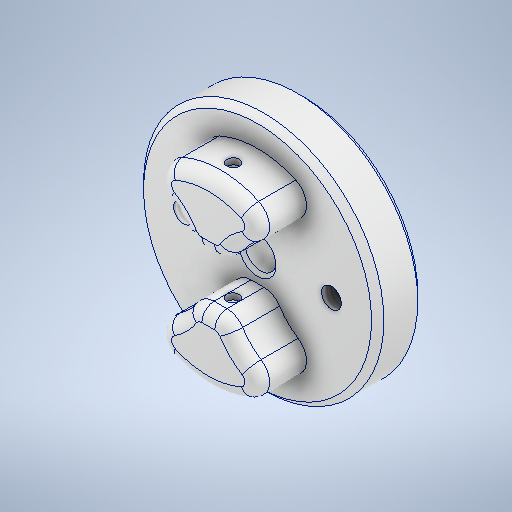
# Autodesk Inventor part: TorquimeterDisk
Saved by Autodesk Inventor 2025 (Build 290162000, 162)
## iProperties
Created: 2024-02-16
Part Number: TorquimeterDisk
Material: Aluminum 6061
Document SubType Name: Modeling
Designer: Vinicius
Density: 2.7 g/cm^3
Appearance: Aluminum - Flat
Mass: 20.646 g
Surface Area: 50.8443 cm^2
Volume: 7.64665 cm^3
Author: Vinicius
Autodesk Inventor part; units mm, degrees
ref_plane "YZ Plane" through (0, 0, 0) normal (1, 0, 0) x (0, 1, 0)
ref_plane "XZ Plane" through (0, 0, 0) normal (0, 1, 0) x (-1, 0, 0)
ref_plane "XY Plane" through (0, 0, 0) normal (0, 0, 1) x (1, 0, 0)
sketch "Sketch1" plane through (0, 0, 0) normal (0, 0, 1) x (1, 0, 0)
  circle A0 centre (0, 0) radius 19.5
  circle A1 centre (0, 0) radius 2.5
  dimension "d0" = 39
  dimension "d1" = 5
  constraints: 2 centre point, 2 coincident
  measures "d0" diameter of A0
  measures "d1" diameter of A1
extrude "Extrusion1" add sketch "Sketch1" along normal blind 7.5
sketch "Sketch2" plane through (0, 0, 7.5) normal (0, 0, 1) x (1, 0, 0)
  point P0 (0, 0)
  point P1 (12, 0)
  point P2 (-12, 0)
  dimension "d4" = 12
  dimension "d5" = 12
  constraints: 2 horizontal alignment
  measures "d4" distance of point (12, 0) point (0, 0)
  measures "d5" distance of point (-12, 0) point (0, 0)
hole "Hole1" at (12, 0, 7.5) at (-12, 0, 7.5) direction (0, 0, -1) diameter 3.242 end through all thread size "M4x0.7" class "6H" standard "ISO Metric profile"
chamfer "Chamfer1" distance 1 angle 45 1 edges at (-19.5, 0, 7.5)
sketch "Sketch5" plane through (0, 0, 7.5) normal (0, 0, 1) x (1, 0, 0)
  circle A0 centre (12, 0) radius 1.621 projected
  circle A1 centre (-12, 0) radius 1.621 projected
  circle A2 centre (12, 0) radius 10
  circle A3 centre (-12, 0) radius 10
  line L0 (2.8348, -4) -> (-2.8348, -4)
  line L1 (2.8348, 4) -> (-2.8348, 4)
  circle A4 centre (0, 0) radius 18.5 projected
  circle A5 centre (0, 0) radius 15
  arc A6 (6.1979, -13.6596) -> (6.5833, -8.4059) centre (4.9583, -10.9277) ccw
  arc A7 (-6.5833, -8.4059) -> (-6.1979, -13.6596) centre (-4.9583, -10.9277) ccw
  arc A8 (-1.0455, -4) -> (-3.5735, -5.3846) centre (-1.0455, -7) ccw
  arc A9 (3.5735, -5.3846) -> (1.0455, -4) centre (1.0455, -7) ccw
  point P0 (0, -4)
  point P1 (0, 4)
  dimension "d26" = 20
  dimension "d27" = 4
  dimension "d28" = 4
  dimension "d29" = 30
  dimension "d30" = 3
  dimension "d31" = 3
  constraints: 18 point on circle, 8 tangent, 7 centre point, 4 end point, 3 equal radius, 2 midpoint, 2 point on line, 1 coincident, 1 horizontal, 1 vertical alignment
  measures "d26" diameter of A3
  measures "d27" distance from line of L1 point (0, 0)
  measures "d28" distance of point (0, -4) point (0, 0)
  measures "d29" diameter of A5
  measures "d30" radius of A6
  measures "d31" radius of A9
extrude "Extrusion2" add sketch "Sketch5" along normal blind 8 contours A2 A6 A5 A7 A3 A8 L0 A9
pattern_circular "Circular Pattern1" count 2 over 360 about axis through (0, 0, 0) along (0, 0, 1) of "Extrusion2"
sketch "Sketch6" plane through (0, 0, 0) normal (0, 1, 0) x (-1, 0, 0)
  circle A0 centre (0, 11.5) radius 1
  line L0 (1.0455, 7.5) -> (1.0455, 15.5) projected
  point P0 (0, 0)
  point P1 (1.0455, 11.5)
  dimension "d37" = 2
  constraints: 1 centre point, 1 horizontal alignment, 1 midpoint, 1 vertical alignment
  measures "d37" diameter of A0
extrude "Extrusion3" cut sketch "Sketch6" along normal through all both and the other way through all
fillet "Fillet2" radius 2 16 edges at (-7.9503, 11.1472, 15.5) (-4.9155, 7.0576, 15.5) (-2.4867, 4.3688, 15.5) (0, 4, 15.5) (2.4867, 4.3688, 15.5) (4.9155, 7.0576, 15.5) (7.9503, 11.1472, 15.5) (0, 15, 15.5) (0, -4, 15.5) (-2.4867, -4.3688, 15.5) (-4.9155, -7.0576, 15.5) (-7.9503, -11.1472, 15.5) (0, -15, 15.5) (7.9503, -11.1472, 15.5) (4.9155, -7.0576, 15.5) (2.4867, -4.3688, 15.5)
sketch "Sketch7" plane through (0, 0, 0) normal (0, 0, -1) x (-1, 0, 0)
  arc A0 (1.0455, 4) -> (3.5735, 5.3846) centre (1.0455, 7) ccw projected
  arc A1 (6.5833, 8.4059) -> (3.5735, 5.3846) centre (12, 0) ccw projected
  arc A2 (6.5833, 8.4059) -> (6.1979, 13.6596) centre (4.9583, 10.9277) ccw projected
  arc A3 (6.1979, 13.6596) -> (-6.1979, 13.6596) centre (0, 0) ccw projected
  arc A4 (-6.1979, 13.6596) -> (-6.5833, 8.4059) centre (-4.9583, 10.9277) ccw projected
  arc A5 (-3.5735, 5.3846) -> (-6.5833, 8.4059) centre (-12, 0) ccw projected
  arc A6 (-3.5735, 5.3846) -> (-1.0455, 4) centre (-1.0455, 7) ccw projected
  line L0 (-1.0455, 4) -> (1.0455, 4) projected
  arc A7 (-1.0455, -4) -> (-3.5735, -5.3846) centre (-1.0455, -7) ccw projected
  arc A8 (-6.5833, -8.4059) -> (-3.5735, -5.3846) centre (-12, 0) ccw projected
  arc A9 (-6.5833, -8.4059) -> (-6.1979, -13.6596) centre (-4.9583, -10.9277) ccw projected
  arc A10 (-6.1979, -13.6596) -> (6.1979, -13.6596) centre (0, 0) ccw projected
  arc A11 (6.1979, -13.6596) -> (6.5833, -8.4059) centre (4.9583, -10.9277) ccw projected
  arc A12 (3.5735, -5.3846) -> (6.5833, -8.4059) centre (12, 0) ccw projected
  arc A13 (3.5735, -5.3846) -> (1.0455, -4) centre (1.0455, -7) ccw projected
  line L1 (1.0455, -4) -> (-1.0455, -4) projected
  circle A14 centre (0, 0) radius 2.5 projected
  circle A15 centre (12, 0) radius 1.621 projected
  circle A16 centre (-12, 0) radius 1.621 projected
  circle A17 centre (0, 0) radius 18.5 projected
  arc A18 (5.7847, 12.749) -> (-5.7847, 12.749) centre (0, 0) ccw
  arc A19 (6.0417, 9.2465) -> (5.7847, 12.749) centre (4.9583, 10.9277) ccw
  arc A20 (6.0417, 9.2465) -> (2.7308, 5.9231) centre (12, 0) ccw
  arc A21 (1.0455, 5) -> (2.7308, 5.9231) centre (1.0455, 7) ccw
  line L2 (1.0455, 5) -> (-1.0455, 5)
  arc A22 (-2.7308, 5.9231) -> (-1.0455, 5) centre (-1.0455, 7) ccw
  arc A23 (-2.7308, 5.9231) -> (-6.0417, 9.2465) centre (-12, 0) ccw
  arc A24 (-5.7847, 12.749) -> (-6.0417, 9.2465) centre (-4.9583, 10.9277) ccw
  arc A25 (-1.0455, -5) -> (-2.7308, -5.9231) centre (-1.0455, -7) ccw
  line L3 (-1.0455, -5) -> (1.0455, -5)
  arc A26 (2.7308, -5.9231) -> (1.0455, -5) centre (1.0455, -7) ccw
  arc A27 (2.7308, -5.9231) -> (6.0417, -9.2465) centre (12, 0) ccw
  arc A28 (5.7847, -12.749) -> (6.0417, -9.2465) centre (4.9583, -10.9277) ccw
  arc A29 (-5.7847, -12.749) -> (5.7847, -12.749) centre (0, 0) ccw
  arc A30 (-6.0417, -9.2465) -> (-5.7847, -12.749) centre (-4.9583, -10.9277) ccw
  arc A31 (-6.0417, -9.2465) -> (-2.7308, -5.9231) centre (-12, 0) ccw
  line L4 (-4.207, 7.7633) -> (4.207, 7.7633)
  line L5 (-4.207, -7.7633) -> (4.207, -7.7633)
  line L6 (-1.0455, 4) -> (-1.0455, 6) projected
  dimension "d41" = 1
  dimension "d42" = 1
  constraints: 32 point on circle, 14 centre point, 8 end point, 1 perpendicular, 14 other
  measures "d41" radial gap between concentric circles of A3 A18
  measures "d42" radial gap between concentric circles of A7 A25
extrude "Extrusion4" cut sketch "Sketch7" against normal blind 14 contours A22 A23 L4 A20 A21 L2 | A23 A24 A18 A19 A20 L4 | L3 A26 A27 L5 A31 A25 | L5 A27 A28 A29 A30 A31
sketch "Sketch8" plane through (0, 0, 0) normal (0, 0, -1) x (-1, 0, 0)
  arc A0 (2.7308, -5.9231) -> (6.0417, -9.2465) centre (12, 0) ccw projected
  arc A1 (5.7847, -12.749) -> (6.0417, -9.2465) centre (4.9583, -10.9277) ccw projected
  arc A2 (-5.7847, -12.749) -> (5.7847, -12.749) centre (0, 0) ccw projected
  arc A3 (-6.0417, -9.2465) -> (-5.7847, -12.749) centre (-4.9583, -10.9277) ccw projected
  arc A4 (-6.0417, -9.2465) -> (-2.7308, -5.9231) centre (-12, 0) ccw projected
  arc A5 (-2.7308, 5.9231) -> (-6.0417, 9.2465) centre (-12, 0) ccw projected
  arc A6 (-5.7847, 12.749) -> (-6.0417, 9.2465) centre (-4.9583, 10.9277) ccw projected
  arc A7 (5.7847, 12.749) -> (-5.7847, 12.749) centre (0, 0) ccw projected
  arc A8 (6.0417, 9.2465) -> (5.7847, 12.749) centre (4.9583, 10.9277) ccw projected
  arc A9 (6.0417, 9.2465) -> (2.7308, 5.9231) centre (12, 0) ccw projected
  circle A10 centre (-12, 0) radius 1.621 projected
  circle A11 centre (12, 0) radius 1.621 projected
  circle A12 centre (0, 0) radius 19.5 projected
  circle A13 centre (0, 0) radius 2.5 projected
  circle A14 centre (0, 0) radius 5
  circle A15 centre (0, 0) radius 8.83
  arc A16 (-4.207, 7.7633) -> (-6.0417, 9.2465) centre (-12, 0) ccw projected
  arc A17 (-5.8433, 6.62) -> (-6.0417, 9.2465) centre (-6.9363, 7.8582) ccw
  arc A18 (6.0417, 9.2465) -> (4.207, 7.7633) centre (12, 0) ccw projected
  arc A19 (6.0417, 9.2465) -> (5.8433, 6.62) centre (6.9363, 7.8582) ccw
  arc A20 (-6.0417, -9.2465) -> (-4.207, -7.7633) centre (-12, 0) ccw projected
  arc A21 (-6.0417, -9.2465) -> (-5.8433, -6.62) centre (-6.9363, -7.8582) ccw
  arc A22 (5.8433, -6.62) -> (6.0417, -9.2465) centre (6.9363, -7.8582) ccw
  arc A23 (-6.0417, -9.2465) -> (-5.7847, -12.749) centre (-4.9583, -10.9277) ccw projected
  arc A24 (2.7308, -5.9231) -> (1.0455, -5) centre (1.0455, -7) ccw projected
  arc A25 (-1.0455, -5) -> (-2.7308, -5.9231) centre (-1.0455, -7) ccw projected
  line L0 (-1.0455, -5) -> (1.0455, -5) projected
  arc A26 (-2.7308, 5.9231) -> (-1.0455, 5) centre (-1.0455, 7) ccw projected
  arc A27 (1.0455, 5) -> (2.7308, 5.9231) centre (1.0455, 7) ccw projected
  line L1 (1.0455, 5) -> (-1.0455, 5) projected
  point P0 (-4.207, -7.7633)
  point P1 (4.207, -7.7633)
  point P2 (-4.207, 7.7633)
  point P3 (4.207, 7.7633)
  dimension "d45" = 10
  constraints: 13 point on circle, 8 tangent, 6 centre point, 2 coincident
  measures "d45" diameter of A14
extrude "Extrusion5" cut sketch "Sketch8" against normal blind 3 contours A24 L0 A14 L1 A27 A9 A15 A0 | A0 A15 A4 A25 L0 A24 | A15 A22 A0 | A15 A5 A26 L1 A14 L0 A25 A4 | A4 A21 A15 | L1 A26 A5 A15 A9 A27 | A17 A5 A15 | A15 A9 A19
sketch "Sketch9" plane through (0, 0, 0) normal (0, 0, -1) x (-1, 0, 0)
  line L0 (0, 6) -> (0, -6) construction
  line L1 (-0.75, 6) -> (-0.75, -6)
  line L2 (0.75, -6) -> (0.75, 6)
  arc A0 (0.75, 6) -> (-0.75, 6) centre (0, 6) ccw
  arc A1 (-0.75, -6) -> (0.75, -6) centre (0, -6) ccw
  point P0 (0, 0)
  dimension "d49" = 6
  dimension "d50" = 1.5
  constraints: 8 end point, 4 point on circle, 4 tangent, 2 centre point, 1 midpoint, 1 parallel, 1 vertical
  measures "d49" distance of point (0, 0) L0.end
  measures "d50" diameter of A1
extrude "Extrusion6" [suppressed]
chamfer "Chamfer2" distance 0.5 angle 45 1 edges at (-2.5, 0, 7.5)
chamfer "Chamfer3" distance 1 angle 45 1 edges at (-19.5, 0, 0)
chamfer "Chamfer4" distance 0.25 angle 45 14 edges at (0, -14, 0) (6.953, -11.074, 0) (5.2894, -7.9826, 0) (8.83, 0, 0) (5.2894, 7.9826, 0) (6.953, 11.074, 0) (0, 14, 0) (-6.953, 11.074, 0) (-5.2894, 7.9826, 0) (-8.83, 0, 0) (-5.2894, -7.9826, 0) (-6.953, -11.074, 0) (5, 0, 0) (-2.5, 0, 0)
equation "\"d5\" = d4"
equation "\"d28\" = d27"
body "Solid1"
